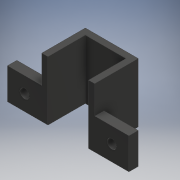
# Autodesk Inventor part: learnbotEncajeMotor
Saved by Autodesk Inventor 2017 (Build 210142000, 142)
## iProperties
Part Number: learnbotEncajeMotor
Material: Genérico
Document SubType Name: Modeling
Designer: rober
Density: 1 g/cm^3
Appearance: Valor por defecto
Author: rober
Autodesk Inventor part; units mm, degrees
ref_plane "YZ Plane" through (0, 0, 0) normal (1, 0, 0) x (0, 1, 0)
ref_plane "XZ Plane" through (0, 0, 0) normal (0, 1, 0) x (-1, 0, 0)
ref_plane "XY Plane" through (0, 0, 0) normal (0, 0, 1) x (1, 0, 0)
sketch "Boceto1" plane through (0, 0, 0) normal (0, 0, 1) x (1, 0, 0)
  line L0 (2.8, 1.4) -> (2.8, 0.3)
  line L1 (2.6, 0) -> (3.9, 0)
  line L2 (3.9, 0) -> (3.9, 0.3)
  line L3 (3.9, 0.3) -> (2.8, 0.3)
  line L4 (0, 0) -> (0, 0.3)
  line L5 (0, 0.3) -> (1.1, 0.3)
  line L6 (0, 0) -> (1.3, 0)
  line L7 (1.3, 0) -> (1.3, 1.2)
  line L8 (2.6, 1.2) -> (2.6, 0)
  line L9 (1.1, 1.4) -> (1.1, 0.3)
  line L10 (1.1, 1.4) -> (2.8, 1.4)
  line L11 (1.3, 1.2) -> (2.6, 1.2)
  constraints: 24 end point
extrude "Extrusión1" add sketch "Boceto1" against normal blind 1
sketch "Boceto2" plane through (0, 0, 0) normal (0, 0, 1) x (1, 0, 0)
  line L0 (1.1, 1.2) -> (2.8, 1.2) projected
  line L1 (1.1, 1.4) -> (1.1, 0.3) projected
  line L2 (2.8, 0.3) -> (2.8, 1.4) projected
  line L3 (1.3, 0) -> (0, 0) projected
  line L4 (1.1, 0) -> (1.3, 0)
  line L5 (1.3, 1.2) -> (1.3, 0) projected
  line L6 (1.3, 0) -> (1.3, 1.2)
  line L7 (2.6, 0) -> (2.6, 1.2) projected
  line L8 (1.3, 1.2) -> (2.6, 1.2)
  line L9 (2.6, 1.2) -> (2.6, 0)
  line L10 (2.6, 0) -> (2.8, 0)
  line L11 (2.8, 1.4) -> (2.8, 0.3) projected
  line L12 (2.8, 0) -> (2.8, 1.4)
  line L13 (1.1, 1.2) -> (2.8, 1.2) projected
  line L14 (2.8, 1.4) -> (1.1, 1.4)
  line L15 (1.1, 1.4) -> (1.1, 0)
  constraints: 16 end point, 7 perpendicular, 1 horizontal, 1 point on line
extrude "Extrusión2" add sketch "Boceto2" along normal blind 0.9
sketch "Boceto3" plane through (2.8, 0.3, 0) normal (0, 1, 0) x (1, 0, 0)
  line L0 (-1.7, 0) -> (-1.7, 1.9)
  line L1 (-1.7, 1.9) -> (0, 1.9)
  line L2 (0, 1.9) -> (0, 0)
  line L3 (0, 0) -> (-1.7, 0)
  line L4 (-1.7, 0) -> (-2.8, 0)
  line L5 (-2.8, 0) -> (-2.8, 1)
  line L6 (-2.8, 1) -> (-1.7, 1)
  line L7 (0, 0) -> (1.1, 0)
  line L8 (1.1, 0) -> (1.1, 1)
  line L9 (1.1, 1) -> (0, 1)
  circle A0 centre (-2.25, 0.5) radius 0.15
  circle A1 centre (0.55, 0.5) radius 0.15
  line L10 (1.1, 0) -> (0, 0) projected
  line L11 (1.1, 0) -> (1.1, 1) projected
  line L12 (0, 1) -> (1.1, 1) projected
  line L13 (0, 0) -> (0, 1) projected
  point P0 (-2.8, 0)
  constraints: 20 end point, 2 centre point, 2 point on line
extrude "Extrusión3" cut sketch "Boceto3" against normal blind 0.9 contours A0 | A1
